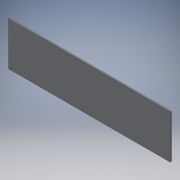
# Autodesk Inventor part: Projector Mount
Saved by Autodesk Inventor 2019 (Build 230136000, 136)
## iProperties
Created: 2020-03-17
Part Number: Projector Mount
Material: Generic
Document SubType Name: Modeling
Designer: Vijay
Density: 1 g/cm^3
Appearance: Default
Author: Vijay
Autodesk Inventor part; units mm, degrees
ref_plane "YZ Plane" through (0, 0, 0) normal (1, 0, 0) x (0, 1, 0)
ref_plane "XZ Plane" through (0, 0, 0) normal (0, 1, 0) x (-1, 0, 0)
ref_plane "XY Plane" through (0, 0, 0) normal (0, 0, 1) x (1, 0, 0)
sketch "Sketch1" plane through (0, 0, 0) normal (0, 0, 1) x (1, 0, 0)
  line L0 (-602, -0.0002) -> (-601.9999, -530.0002) construction
  line L1 (28, -530) -> (28, 100) construction
  line L2 (-582.9, 99.9998) -> (-582.8999, -530.0002) construction
  line L3 (-591.1, 99.9998) -> (-582.9, 99.9998) construction
  line L4 (-591.1, 99.9998) -> (-591.0999, -530.0002) construction
  line L5 (-582.8999, -530.0002) -> (-591.0999, -530.0002) construction
  line L6 (17.1, 100) -> (17.1, -530) construction
  line L7 (8.9, 100) -> (17.1, 100) construction
  line L8 (8.9, 100) -> (8.9, -530) construction
  line L9 (17.1, -530) -> (8.9, -530) construction
  line L10 (13, -530) -> (13, 100) construction
  line L11 (-586.9999, -530.0002) -> (-587, 99.9998) construction
  line L12 (-601.9999, -491.9214) -> (28, -491.9214)
  line L13 (28, -491.9214) -> (28, -321.9214)
  line L14 (28, -321.9214) -> (-601.9999, -321.9214)
  line L15 (-601.9999, -321.9214) -> (-601.9999, -491.9214)
  circle A0 centre (-586.9999, -481.9214) radius 2.5
  circle A1 centre (-586.9999, -331.9214) radius 2.5
  circle A2 centre (13, -481.9214) radius 2.5
  circle A3 centre (13, -331.9214) radius 2.5
  point P0 (0, 0)
  dimension "d0" = 170
  dimension "d1" = 5
  dimension "d2" = 5
  dimension "d3" = 5
  dimension "d4" = 5
  dimension "d5" = 10
  dimension "d6" = 10
  dimension "d7" = 10
  dimension "d8" = 10
  constraints: 14 end point, 6 point on line, 4 centre point, 4 midpoint, 2 parallel, 1 horizontal, 1 perpendicular, 1 vertical, 2 other
  measures "d0" distance between parallel lines of L12 L14
  measures "d1" diameter of A0
  measures "d2" diameter of A1
  measures "d3" diameter of A2
  measures "d4" diameter of A3
  measures "d5" distance from line of L12 A0.centre
  measures "d6" distance from line of L14 A1.centre
  measures "d7" distance from line of A2.centre L12
  measures "d8" distance from line of L14 A3.centre
extrude "Extrusion1" add sketch "Sketch1" along normal blind 4
fillet "Fillet1" radius 2 4 edges at (28, -491.9214, 2) (28, -321.9214, 2) (-601.9999, -321.9214, 2) (-601.9999, -491.9214, 2)
body "Solid1"
